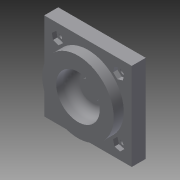
# Autodesk Inventor part: BallBearingCupMount
Saved by Autodesk Inventor 2015 (Build 190159000, 159)
## iProperties
Created: 2017-01-13
Part Number: BallBearingCupMount
Material: Generic
Document SubType Name: Modeling
Designer: 1esh9
Density: 1 g/cm^3
Appearance: Default
Author: 1esh9
Autodesk Inventor part; units mm, degrees
ref_plane "YZ Plane" through (0, 0, 0) normal (1, 0, 0) x (0, 1, 0)
ref_plane "XZ Plane" through (0, 0, 0) normal (0, 1, 0) x (-1, 0, 0)
ref_plane "XY Plane" through (0, 0, 0) normal (0, 0, 1) x (1, 0, 0)
sketch "Sketch1" plane through (0, 0, 0) normal (0, 0, 1) x (1, 0, 0)
  line L0 (0, -8.6) -> (12.34, -8.6) construction
  line L1 (0, 0) -> (0, -8.6)
  line L2 (0, 0) -> (0, -2.1)
  line L3 (0, -2.1) -> (5.3, -2.1)
  line L4 (5.3, -2.1) -> (5.3, 0)
  line L5 (5.3, 0) -> (7.44, 0)
  line L6 (12.44, -8.7) -> (12.44, -5)
  arc A0 (12.44, -5) -> (7.44, 0) centre (7.44, -5) ccw
  line L7 (12.44, -8.7) -> (20.44, -8.7)
  line L8 (20.44, -8.7) -> (20.44, 5)
  line L9 (20.44, 5) -> (0, 5)
  line L10 (0, 5) -> (0, -2.1)
  line L11 (-4.088, 0) -> (24.528, 0) projected
  dimension "d2" = 12.34
  dimension "d3" = 8.6
  dimension "d7" = 0
  dimension "d11" = 5.3
  dimension "d12" = 2.1
  dimension "d14" = 5
  dimension "d15" = 8
  dimension "d16" = 13.7
  dimension "d17" = 3.7
  dimension "d18" = 5
  constraints: 22 end point, 4 perpendicular, 2 collinear, 2 horizontal, 2 point on circle, 2 tangent, 1 centre point, 1 point on line, 1 vertical
  measures "d2" distance of L0.start L0.end
  measures "d3" distance from line of L0 L1.start
  measures "d7" horizontal distance of L1.start L0.start
  measures "d11" distance of L2.end L3.end
  measures "d12" distance of L3.end L4.end
  measures "d14" radius of A0
  measures "d15" distance of L6.start L7.end
  measures "d16" distance of L7.end L8.end
  measures "d17" distance of L6.start L6.end
  measures "d18" distance between parallel lines of L9 L11
revolve "Revolution2" add sketch "Sketch1" angle 360 about axis through (0, 5, 0) along (0, -1, 0)
sketch "Sketch2" plane through (0, 5, 0) normal (0, 1, 0) x (1, 0, 0)
  line L0 (-25, 25) -> (25, 25)
  line L1 (25, 25) -> (25, -25)
  line L2 (25, -25) -> (-25, -25)
  line L3 (-25, -25) -> (-25, 25)
  line L4 (-17.5, 17.5) -> (17.5, 17.5) construction
  line L5 (17.5, 17.5) -> (17.5, -17.5) construction
  line L6 (17.5, -17.5) -> (-17.5, -17.5) construction
  line L7 (-17.5, -17.5) -> (-17.5, 17.5) construction
  circle A0 centre (-17.5, 17.5) radius 1.7
  circle A1 centre (17.5, 17.5) radius 1.7
  circle A2 centre (-17.5, -17.5) radius 1.7
  circle A3 centre (17.5, -17.5) radius 1.7
  line L8 (18.3404, 20.6818) -> (20.6757, 18.3631)
  line L9 (20.6757, 18.3631) -> (19.8353, 15.1813)
  line L10 (19.8353, 15.1813) -> (16.6596, 14.3182)
  line L11 (16.6596, 14.3182) -> (14.3243, 16.6369)
  line L12 (14.3243, 16.6369) -> (15.1647, 19.8187)
  line L13 (15.1647, 19.8187) -> (18.3404, 20.6818)
  line L14 (-16.6058, 14.3329) -> (-19.7956, 15.142)
  line L15 (-19.7956, 15.142) -> (-20.6899, 18.3091)
  line L16 (-20.6899, 18.3091) -> (-18.3942, 20.6671)
  line L17 (-18.3942, 20.6671) -> (-15.2044, 19.858)
  line L18 (-15.2044, 19.858) -> (-14.3101, 16.6909)
  line L19 (-14.3101, 16.6909) -> (-16.6058, 14.3329)
  line L20 (-15.0239, -19.6677) -> (-18.1393, -20.7282)
  line L21 (-18.1393, -20.7282) -> (-20.6153, -18.5605)
  line L22 (-20.6153, -18.5605) -> (-19.9761, -15.3323)
  line L23 (-19.9761, -15.3323) -> (-16.8607, -14.2718)
  line L24 (-16.8607, -14.2718) -> (-14.3847, -16.4395)
  line L25 (-14.3847, -16.4395) -> (-15.0239, -19.6677)
  line L26 (19.9241, -15.2743) -> (20.6396, -18.4864)
  line L27 (20.6396, -18.4864) -> (18.2155, -20.7122)
  line L28 (18.2155, -20.7122) -> (15.0759, -19.7257)
  line L29 (15.0759, -19.7257) -> (14.3604, -16.5136)
  line L30 (14.3604, -16.5136) -> (16.7845, -14.2878)
  line L31 (16.7845, -14.2878) -> (19.9241, -15.2743)
  circle A4 centre (0, 0) radius 12.44 projected
  circle A5 centre (0, 0) radius 12.44 projected
  point P0 (17.5, 17.5)
  dimension "d25" = 35
  dimension "d27" = 17.5
  dimension "d28" = 17.5
  dimension "d29" = 35
  dimension "d30" = 3.4
  dimension "d31" = 3.4
  dimension "d32" = 3.4
  dimension "d33" = 3.4
  dimension "d34" = 5.7
  dimension "d36" = 5.7
  dimension "d37" = 5.7
  dimension "d38" = 5.7
  dimension "d39" = 50
  dimension "d40" = 50
  dimension "d41" = 25
  dimension "d42" = 25
  constraints: 64 end point, 8 coincident, 4 centre point, 4 parallel, 2 horizontal, 2 perpendicular, 52 other
  measures "d25" distance of L5.end L6.end
  measures "d27" distance from line of point (0, 0) L7
  measures "d28" distance from line of L4 point (0, 0)
  measures "d29" distance between parallel lines of L4 L6
  measures "d30" diameter of A0
  measures "d31" diameter of A1
  measures "d32" diameter of A2
  measures "d33" diameter of A3
  measures "d34" distance between parallel lines of L27 L30
  measures "d36" distance between parallel lines of L11 L8
  measures "d37" distance between parallel lines of L16 L19
  measures "d38" distance between parallel lines of L22 L25
  measures "d39" distance of L0.start L0.end
  measures "d40" distance of L2.end L0.start
  measures "d41" distance from line of L3 point (0, 0)
  measures "d42" distance from line of point (0, 0) L0
extrude "Extrusion1" add sketch "Sketch2" against normal blind 8 contours L0 L1 L2 L3
extrude "Extrusion2" add sketch "Sketch2" against normal blind 5.5 contours L8 L9 L10 L11 L12 L13 | L14 L15 L16 L17 L18 L19 | L20 L21 L22 L23 L24 L25 | L26 L27 L28 L29 L30 L31
equation "\"d27\" = 0.5 * d29"
equation "\"d28\" = d27"
equation "\"d36\" = d34"
equation "\"d37\" = d34"
equation "\"d38\" = d34"
equation "\"d41\" = 0.5 * d39"
equation "\"d42\" = d41"
body "Solid2"
